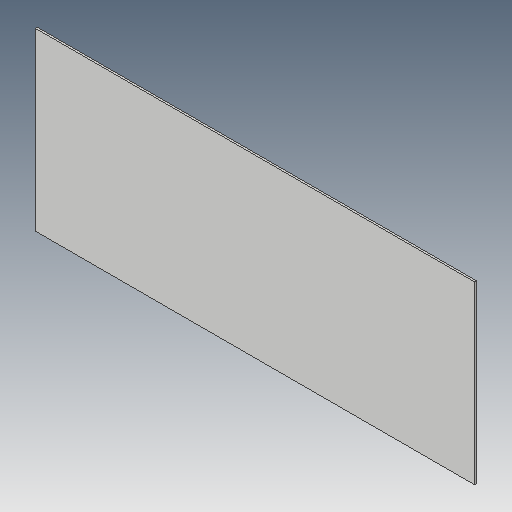
# Autodesk Inventor part: BackVerticalMount
Saved by Autodesk Inventor 2017 (Build 210142000, 142)
## iProperties
Created: 2017-05-22
Part Number: BackVerticalMount
Material: Generic
Document SubType Name: Modeling
Designer: krosie
Density: 1 g/cm^3
Appearance: Default
Author: krosie
Autodesk Inventor part; units mm, degrees
ref_plane "YZ Plane" through (0, 0, 0) normal (1, 0, 0) x (0, 1, 0)
ref_plane "XZ Plane" through (0, 0, 0) normal (0, 1, 0) x (-1, 0, 0)
ref_plane "XY Plane" through (0, 0, 0) normal (0, 0, 1) x (1, 0, 0)
sketch "Sketch1" plane through (0, 0, 0) normal (0, 0, 1) x (1, 0, 0)
  line L0 (-34, 0) -> (-34, 110) projected
  line L1 (416, 110) -> (416, 0) projected
  line L2 (886, 110) -> (886, 0) projected
  line L3 (-504, 0) -> (-504, 110) projected
  line L4 (-34, 110) -> (416, 110)
  line L5 (416, 110) -> (416, -70)
  line L6 (416, -70) -> (-34, -70)
  line L7 (-34, -70) -> (-34, 110)
  dimension "d0" = 180
  constraints: 8 end point, 2 parallel, 1 horizontal, 1 perpendicular, 1 point on line
  measures "d0" distance of L4.end L5.end
extrude "Extrusion1" add sketch "Sketch1" along normal blind 2
body "Solid1"
